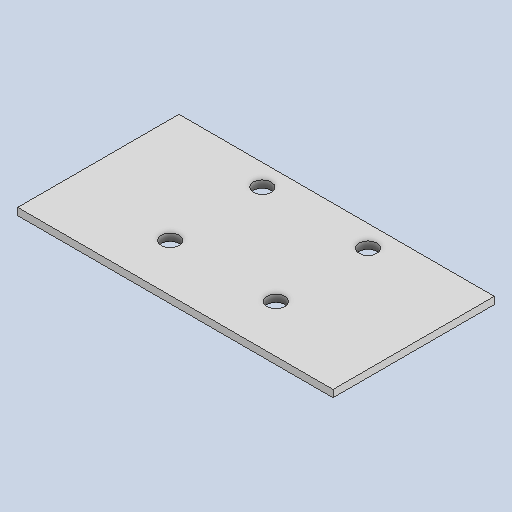
# Autodesk Inventor part: PlacaSTC-HH20
Saved by Autodesk Inventor 2022 (Build 260153000, 153)
## iProperties
Created: 2022-03-28
Part Number: PlacaSTC-HH20
Material: Genérico
Document SubType Name: Modeling
Designer: aarco
Density: 1 g/cm^3
Appearance: Valor por defecto
Author: aarco
Autodesk Inventor part; units mm, degrees
ref_plane "YZ Plane" through (0, 0, 0) normal (1, 0, 0) x (0, 1, 0)
ref_plane "XZ Plane" through (0, 0, 0) normal (0, 1, 0) x (-1, 0, 0)
ref_plane "XY Plane" through (0, 0, 0) normal (0, 0, 1) x (1, 0, 0)
sketch "Boceto1" plane through (0, 0, 0) normal (0, 1, 0) x (-1, 0, 0)
  line L0 (44, 22.5) -> (-44, 22.5)
  line L1 (-44, 22.5) -> (-44, -22.5)
  line L2 (-44, -22.5) -> (44, -22.5)
  line L3 (44, -22.5) -> (44, 22.5)
  line L4 (44, 22.5) -> (-44, -22.5) construction
  circle A0 centre (14.75, -16.5) radius 2.5
  circle A1 centre (14.75, 9.2) radius 2.5
  line L5 (14.75, -16.5) -> (-14.75, -16.5) construction
  line L6 (-14.75, -16.5) -> (-14.75, 9.2) construction
  line L7 (-14.75, 9.2) -> (14.75, 9.2) construction
  line L8 (14.75, 9.2) -> (14.75, -16.5) construction
  line L9 (0, 0) -> (0, -30.1177)
  circle A2 centre (-14.75, -16.5) radius 2.5
  circle A3 centre (-14.75, 9.2) radius 2.5
  dimension "d0" = 88
  dimension "d1" = 45
  dimension "d4" = 5
  dimension "d5" = 25.7
  dimension "d6" = 6
  dimension "d7" = 29.5
  constraints: 20 end point, 4 centre point, 4 coincident, 4 parallel, 3 equal radius, 2 horizontal, 2 perpendicular, 1 midpoint, 1 symmetric about line, 1 vertical
  measures "d0" distance of L0.start L0.end
  measures "d1" distance of L2.end L0.start
  measures "d4" diameter of A0
  measures "d5" distance of L7.end L5.start
  measures "d6" distance between parallel lines of L2 L5
  measures "d7" distance of L5.start L5.end
extrude "Extrusión1" add sketch "Boceto1" along normal blind 2
